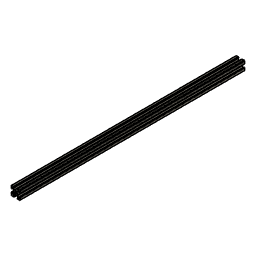
2020-extrusion (Autodesk Fusion 360 design; units mm, degrees)
Autodesk Fusion 360 part; units mm, degrees
sketch "Sketch1" plane through (0, 0, 0) normal (0, 1, 0) x (1, 0, 0)
  line L0 (9, -10) -> (-9, -10)
  line L1 (-10, -9) -> (-10, 9)
  line L2 (-9, 10) -> (9, 10)
  line L3 (10, 9) -> (10, -9)
  line L4 (10, -10) -> (-10, 10) construction
  line L5 (-10, -10) -> (10, 10) construction
  line L6 (4, -4) -> (-4, -4)
  line L7 (-4, -4) -> (-4, 4)
  line L8 (-4, 4) -> (4, 4)
  line L9 (4, 4) -> (4, -4)
  line L10 (4, -4) -> (-4, 4) construction
  line L11 (-4, -4) -> (4, 4) construction
  circle A0 centre (0, 0) radius 2
  line L12 (8.45, -8.45) -> (-8.45, -8.45)
  line L13 (-8.45, -8.45) -> (-8.45, 8.45)
  line L14 (-8.45, 8.45) -> (8.45, 8.45)
  line L15 (8.45, 8.45) -> (8.45, -8.45)
  line L16 (8.45, -8.45) -> (-8.45, 8.45) construction
  line L17 (-8.45, -8.45) -> (8.45, 8.45) construction
  line L18 (-9.452, -10.548) -> (10.548, 9.452) construction
  line L19 (-10.548, -9.452) -> (9.452, 10.548) construction
  line L20 (10.548, -9.452) -> (-9.452, 10.548) construction
  line L21 (9.452, -10.548) -> (-10.548, 9.452) construction
  line L22 (3.1, -10) -> (-3.1, -10) construction
  line L23 (-3.1, -10) -> (-3.1, 10) construction
  line L24 (-3.1, 10) -> (3.1, 10) construction
  line L25 (3.1, 10) -> (3.1, -10) construction
  line L26 (10, -3.1) -> (-10, -3.1) construction
  line L27 (-10, -3.1) -> (-10, 3.1) construction
  line L28 (-10, 3.1) -> (10, 3.1) construction
  line L29 (10, 3.1) -> (10, -3.1) construction
  line L30 (-3.1, -8.45) -> (-3.1, -10)
  line L31 (3.1, -8.45) -> (3.1, -10)
  line L32 (-8.45, -3.1) -> (-10, -3.1)
  line L33 (-8.45, 3.1) -> (-10, 3.1)
  line L34 (8.45, -3.1) -> (10, -3.1)
  line L35 (8.45, 3.1) -> (10, 3.1)
  line L36 (-3.1, 8.45) -> (-3.1, 10)
  line L37 (3.1, 8.45) -> (3.1, 10)
  line L38 (-4, 2.904) -> (-8.45, 7.354)
  line L39 (-2.904, 4) -> (-7.354, 8.45)
  line L40 (2.904, 4) -> (7.354, 8.45)
  line L41 (4, 2.904) -> (8.45, 7.354)
  line L42 (-4, -2.904) -> (-8.45, -7.354)
  line L43 (-2.904, -4) -> (-7.354, -8.45)
  line L44 (2.904, -4) -> (7.354, -8.45)
  line L45 (4, -2.904) -> (8.45, -7.354)
  line L46 (-10, -3.1) -> (-9.55, -3.1)
  line L47 (-9.55, -3.1) -> (-9.55, -3.6)
  line L48 (-9.55, -3.6) -> (-10, -3.6)
  line L49 (-10, -3.6) -> (-10, -3.1)
  line L50 (-10, 3.1) -> (-9.55, 3.1)
  line L51 (-9.55, 3.1) -> (-9.55, 3.6)
  line L52 (-9.55, 3.6) -> (-10, 3.6)
  line L53 (-10, 3.6) -> (-10, 3.1)
  line L54 (-3.1, -10) -> (-3.6, -10)
  line L55 (-3.6, -10) -> (-3.6, -9.55)
  line L56 (-3.6, -9.55) -> (-3.1, -9.55)
  line L57 (-3.1, -9.55) -> (-3.1, -10)
  line L58 (3.1, -10) -> (3.6, -10)
  line L59 (3.6, -10) -> (3.6, -9.55)
  line L60 (3.6, -9.55) -> (3.1, -9.55)
  line L61 (3.1, -9.55) -> (3.1, -10)
  line L62 (10, -3.1) -> (9.55, -3.1)
  line L63 (9.55, -3.1) -> (9.55, -3.6)
  line L64 (9.55, -3.6) -> (10, -3.6)
  line L65 (10, -3.6) -> (10, -3.1)
  line L66 (10, 3.1) -> (9.55, 3.1)
  line L67 (9.55, 3.1) -> (9.55, 3.6)
  line L68 (9.55, 3.6) -> (10, 3.6)
  line L69 (10, 3.6) -> (10, 3.1)
  line L70 (-3.1, 10) -> (-3.6, 10)
  line L71 (-3.6, 10) -> (-3.6, 9.55)
  line L72 (-3.6, 9.55) -> (-3.1, 9.55)
  line L73 (-3.1, 9.55) -> (-3.1, 10)
  line L74 (3.1, 10) -> (3.55, 10)
  line L75 (3.55, 10) -> (3.55, 9.5)
  line L76 (3.55, 9.5) -> (3.1, 9.5)
  line L77 (3.1, 9.5) -> (3.1, 10)
  arc A1 (-10, -9) -> (-9, -10) centre (-9, -9) ccw
  arc A2 (9, -10) -> (10, -9) centre (9, -9) ccw
  arc A3 (10, 9) -> (9, 10) centre (9, 9) ccw
  arc A4 (-9, 10) -> (-10, 9) centre (-9, 9) ccw
  dimension "d1" = 20
  dimension "d2" = 20
  dimension "d3" = 8
  dimension "d4" = 8
  dimension "d5" = 4
  dimension "d6" = 16.9
  dimension "d7" = 16.9
  dimension "d8" = 0.775
  dimension "d9" = -0.775
  dimension "d10" = 0.775
  dimension "d11" = -0.775
  dimension "d12" = 6.2
  dimension "d13" = 20
  dimension "d14" = 20
  dimension "d15" = 6.2
  dimension "d16" = 1.55
  dimension "d17" = 1.55
  dimension "d18" = 1.55
  dimension "d19" = 1.55
  dimension "d20" = 1.55
  dimension "d21" = 1.55
  dimension "d22" = 1.55
  dimension "d23" = 1.55
  dimension "d24" = 0.45
  dimension "d25" = 0.5
  dimension "d26" = 0.45
  dimension "d27" = 0.5
  dimension "d28" = 0.5
  dimension "d29" = 0.45
  dimension "d30" = 0.5
  dimension "d31" = 0.45
  dimension "d32" = 0.45
  dimension "d33" = 0.5
  dimension "d34" = 0.45
  dimension "d35" = 0.5
  dimension "d36" = 0.5
  dimension "d37" = 0.45
  dimension "d38" = 0.45
  dimension "d39" = 0.5
  dimension "d40" = 1
  dimension "d41" = 1
  dimension "d42" = 1
  dimension "d43" = 1
  constraint horizontal L0
  constraint perpendicular L0 L1
  constraint parallel L0 L2
  constraint parallel L1 L3
  constraint coincident L4 A0.centre
  constraint coincident L5 A0.centre
  constraint coincident A0.centre origin
  constraint horizontal L6
  constraint perpendicular L6 L7
  constraint parallel L6 L8
  constraint parallel L7 L9
  constraint coincident L10 A0.centre
  constraint coincident L11 A0.centre
  constraint horizontal L12
  constraint perpendicular L12 L13
  constraint parallel L12 L14
  constraint parallel L13 L15
  constraint coincident L16 A0.centre
  constraint coincident L17 A0.centre
  constraint horizontal L22
  constraint perpendicular L22 L23
  constraint parallel L22 L24
  constraint parallel L23 L25
  constraint horizontal L26
  constraint perpendicular L26 L27
  constraint parallel L26 L28
  constraint parallel L27 L29
  constraint vertical L30
  constraint coincident L23 L30.start
  constraint coincident L12 L30.start
  constraint vertical L31
  constraint coincident L12 L31.start
  constraint coincident L25 L31.start
  constraint horizontal L32
  constraint coincident L13 L32.start
  constraint coincident L26 L32.start
  constraint horizontal L33
  constraint coincident L13 L33.start
  constraint coincident L28 L33.start
  constraint horizontal L34
  constraint coincident L15 L34.start
  constraint coincident L26 L34.start
  constraint coincident L28 L35.start
  constraint coincident L15 L35.start
  constraint perpendicular L3 L35
  constraint vertical L36
  constraint coincident L14 L36.start
  constraint coincident L23 L36.start
  constraint vertical L37
  constraint coincident L14 L37.start
  constraint coincident L25 L37.start
  constraint coincident L21 L38.start
  constraint coincident L7 L38.start
  constraint coincident L21 L38.end
  constraint coincident L13 L38.end
  constraint coincident L8 L39.start
  constraint coincident L20 L39.start
  constraint coincident L14 L39.end
  constraint coincident L20 L39.end
  constraint coincident L8 L40.start
  constraint coincident L19 L40.start
  constraint coincident L19 L40.end
  constraint coincident L14 L40.end
  constraint coincident L18 L41.start
  constraint coincident L9 L41.start
  constraint coincident L18 L41.end
  constraint coincident L15 L41.end
  constraint coincident L7 L42.start
  constraint coincident L19 L42.start
  constraint coincident L19 L42.end
  constraint coincident L13 L42.end
  constraint coincident L18 L43.start
  constraint coincident L6 L43.start
  constraint coincident L18 L43.end
  constraint coincident L12 L43.end
  constraint coincident L6 L44.start
  constraint coincident L21 L44.start
  constraint coincident L12 L44.end
  constraint coincident L21 L44.end
  constraint coincident L9 L45.start
  constraint coincident L20 L45.start
  constraint coincident L20 L45.end
  constraint coincident L15 L45.end
  constraint horizontal L46
  constraint vertical L47
  constraint horizontal L48
  constraint vertical L49
  constraint horizontal L50
  constraint vertical L51
  constraint horizontal L52
  constraint vertical L53
  constraint horizontal L54
  constraint vertical L55
  constraint horizontal L56
  constraint vertical L57
  constraint horizontal L58
  constraint vertical L59
  constraint horizontal L60
  constraint vertical L61
  constraint horizontal L62
  constraint vertical L63
  constraint horizontal L64
  constraint vertical L65
  constraint horizontal L66
  constraint vertical L67
  constraint horizontal L68
  constraint vertical L69
  constraint horizontal L70
  constraint vertical L71
  constraint horizontal L72
  constraint vertical L73
  constraint horizontal L74
  constraint vertical L75
  constraint horizontal L76
  constraint vertical L77
  constraint coincident L5.start L0
  constraint coincident L5.start L1
  constraint tangent L0 A1
  constraint tangent L1 A1
  constraint coincident L4.start L0
  constraint coincident L4.start L3
  constraint tangent L0 A2
  constraint tangent L3 A2
  constraint coincident L5.end L3
  constraint coincident L5.end L2
  constraint tangent L3 A3
  constraint tangent L2 A3
  constraint coincident L4.end L2
  constraint coincident L4.end L1
  constraint tangent L2 A4
  constraint tangent L1 A4
  measures "d1" distance of L4.end L5.end
  measures "d2" distance of L5.start L4.end
  measures "d3" distance of L7.end L8.end
  measures "d4" distance of L6.end L7.end
  measures "d5" diameter of A0
  measures "d6" distance of L13.end L14.end
  measures "d7" distance of L12.end L13.end
  measures "d12" distance of L23.end L24.end
  measures "d13" distance of L22.end L23.end
  measures "d14" distance of L27.end L28.end
  measures "d15" distance of L26.end L27.end
  measures "d16" distance of L30.start L22.end
  measures "d17" distance of L31.start L22.start
  measures "d18" distance of L32.start L26.end
  measures "d19" distance of L33.start L27.end
  measures "d20" distance of L34.start L26.start
  measures "d21" distance of L35.start L28.end
  measures "d22" distance of L36.start L23.end
  measures "d23" distance of L37.start L24.end
  measures "d24" distance of L26.end L46.end
  measures "d25" distance of L26.end L48.end
  measures "d26" distance of L27.end L50.end
  measures "d27" distance of L27.end L52.end
  measures "d28" distance of L22.end L54.end
  measures "d29" distance of L22.end L56.end
  measures "d30" distance of L22.start L58.end
  measures "d31" distance of L22.start L60.end
  measures "d32" distance of L26.start L62.end
  measures "d33" distance of L26.start L64.end
  measures "d34" distance of L28.end L66.end
  measures "d35" distance of L28.end L68.end
  measures "d36" distance of L23.end L70.end
  measures "d37" distance of L23.end L72.end
  measures "d38" distance of L24.end L74.end
  measures "d39" distance of L24.end L76.end
  measures "d40" radius of A1
  measures "d41" radius of A2
  measures "d42" radius of A3
  measures "d43" radius of A4
extrude "Extrude1" add sketch "Sketch1" along normal blind 500 contours L0 L3 L12 L15 L31 L34 L59 L60 L63 L64 A2 | L0 L1 L12 L13 L30 L32 L47 L48 L55 L56 A1 | L6 L9 L12 L15 L44 L45 | L2 L3 L14 L15 L35 L37 L67 L68 L75 L76 A3 | L6 L7 L12 L13 L42 L43 | L6 L7 L8 L9 | L8 L9 L14 L15 L40 L41 | L1 L2 L13 L14 L33 L36 L51 L52 L71 L72 A4 | L7 L8 L13 L14 L38 L39
fillet "Fillet1" radius 0.5 16 edges at (-8.45, 250, -7.354) (-7.354, 250, -8.45) (7.354, 250, -8.45) (8.45, 250, -7.354) (8.45, 250, 7.354) (7.354, 250, 8.45) (-7.354, 250, 8.45) (-8.45, 250, 7.354) (-2.904, 250, 4) (2.904, 250, 4) (-4, 250, 2.904) (-4, 250, -2.904) (-2.904, 250, -4) (2.904, 250, -4) (4, 250, -2.904) (4, 250, 2.904)
equation "d6 = 20 mm - ( ( 1.55 * 2 ) * 1 mm )"
equation "d7 = 20 mm - ( ( 1.55 * 2 ) * 1 mm )"
equation "d8 = ( 1.55 / 2 ) * 1 mm"
equation "d9 = ( -1.55 / 2 ) * 1 mm"
equation "d10 = ( 1.55 / 2 ) * 1 mm"
equation "d11 = ( -1.55 / 2 ) * 1 mm"
named bodies: "2020-extrusion"
